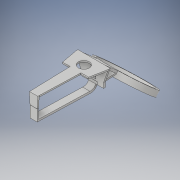
# Autodesk Inventor part: WesRoboticsInvention2019
Saved by Autodesk Inventor 2017 (Build 210142000, 142)
## iProperties
Created: 2019-11-21
Part Number: WesRoboticsInvention2019
Material: Generic
Document SubType Name: Modeling
Designer: Wes
Density: 1 g/cm^3
Appearance: Default
Author: Wes
Autodesk Inventor part; units mm, degrees
ref_plane "YZ Plane" through (0, 0, 0) normal (1, 0, 0) x (0, 1, 0)
ref_plane "XZ Plane" through (0, 0, 0) normal (0, 1, 0) x (-1, 0, 0)
ref_plane "XY Plane" through (0, 0, 0) normal (0, 0, 1) x (1, 0, 0)
sketch "sketch1 - front_main" plane through (0, 0, 0) normal (0, 0, 1) x (1, 0, 0)
  line L0 (0, 0.4311) -> (0, 247.3755) construction
  line L1 (0, 247.3755) -> (246.9445, 247.3755) construction
  line L2 (246.9445, 247.3755) -> (246.9445, 0.4311) construction
  line L3 (246.9445, 0.4311) -> (0, 0.4311) construction
  line L4 (150.2802, 116.2764) -> (77.9266, 114.0849)
  line L5 (77.9266, 114.0849) -> (77.9266, 100.4804)
  line L6 (77.9266, 100.4804) -> (48.3439, 94.9879)
  line L7 (150.2802, 131.1589) -> (77.9266, 133.3504)
  line L8 (77.9266, 133.3504) -> (77.9266, 146.9549)
  line L9 (77.9266, 146.9549) -> (48.3439, 152.4474)
  line L10 (150.2802, 116.2764) -> (150.2802, 131.1589)
  line L11 (48.3439, 94.9879) -> (48.3439, 152.4474)
  circle A0 centre (63.1352, 123.7176) radius 9.6612
  point P0 (0, 0)
  constraints: 16 end point, 1 centre point, 1 vertical, 2 other
extrude "Extrusion2" add sketch "sketch1 - front_main" along normal blind 2.5 contours L4 L5 L6 L11 L9 L8 L7 L10 | A0
sketch "sketch2 - bottom_front_tab" plane through (150.2802, 116.2764, 0) normal (1, 0, 0) x (0, 0, -1)
  line L0 (-2.5, 0) -> (-2.5, 14.8824)
  line L1 (-2.5, 0) -> (17.4726, 1.0467)
  line L2 (-2.5, 14.8824) -> (17.4726, 13.8357)
  line L3 (17.4726, 13.8357) -> (17.4726, 1.0467)
  point P0 (0, -116.2764)
  dimension "d14" = 20
  dimension "d16" = 20
  constraints: 8 end point
  measures "d14" distance of L0.start L1.end
  measures "d16" distance of L0.end L2.end
extrude "Extrusion3" add sketch "sketch2 - bottom_front_tab" along normal blind 2.5
sketch "sketch3 - top_tab" plane through (48.3439, 94.9879, 0) normal (-1, 0, 0) x (0, 0, 1)
  line L0 (30.1774, 130.7193) -> (30.1774, -83.6008) construction
  line L1 (30.1774, -83.6008) -> (-73.7679, -83.6008) construction
  line L2 (-73.7679, -83.6008) -> (-73.7679, 130.7193) construction
  line L3 (-73.7679, 130.7193) -> (30.1774, 130.7193) construction
  line L4 (2.5, 0) -> (2.5, 5.4925) projected
  line L5 (2.5, 57.4594) -> (2.5, 0)
  line L6 (2.5, 0) -> (-22.0835, 8.4648)
  line L7 (2.5, 57.4594) -> (2.5, 0) projected
  line L8 (2.5, 57.4594) -> (-22.0835, 48.9947)
  line L9 (2.5, 57.4594) -> (28.5, 57.4594) construction
  line L10 (-22.0835, 48.9947) -> (-31.0835, 48.9947)
  line L11 (-31.0835, 8.4648) -> (-22.0835, 8.4648)
  line L12 (-23.2529, 28.8344) -> (-23.2529, 35.3344)
  line L13 (-23.2529, 35.3344) -> (-17.4726, 35.1242)
  line L14 (-23.2529, 28.8344) -> (-23.2529, 22.3344)
  line L15 (-17.4726, 22.3352) -> (-17.4726, 35.1242) projected
  line L16 (-17.4726, 35.1242) -> (-17.4726, 22.3352)
  line L17 (-17.4726, 22.3352) -> (-23.2529, 22.3344)
  line L18 (-31.0835, 37.7297) -> (-31.0835, 48.9947)
  line L19 (-31.0835, 19.7297) -> (-31.0835, 8.4648)
  line L20 (-31.0835, 19.7297) -> (-26.3187, 19.7297)
  line L21 (-26.3187, 19.7297) -> (-26.3187, 37.7297)
  line L22 (-26.3187, 37.7297) -> (-31.0835, 37.7297)
  dimension "d66" = 26
  dimension "d67" = 71
  dimension "d68" = 26
  dimension "d69" = 161
  dimension "d70" = 9
  dimension "d73" = 6.5
  dimension "d74" = 6.5
  constraints: 32 end point, 4 horizontal, 2 collinear, 2 vertical, 1 equal length, 1 perpendicular, 2 other
  measures "d66" distance of L4.start L6.end
  measures "d67" angle of L5 L6
  measures "d68" distance of L5.start L8.end
  measures "d69" angle of L8 L9
  measures "d70" distance of L8.end L10.end
  measures "d73" distance of L12.start L12.end
  measures "d74" distance of L12.start L14.end
extrude "Extrusion5" add sketch "sketch3 - top_tab" along normal blind 3.5
ref_plane "Work Plane1" through (203.0833, 123.7176, 2.5) normal (0, 1, 0) x (0, 0, 1)
sketch "sketch4 - xbox_hole" plane through (0, 0, 2.5) normal (0, 0, 1) x (1, 0, 0)
  circle A0 centre (63.1352, 123.7176) radius 9.6612
  point P0 (0, 0)
  constraints: 1 centre point
extrude "Extrusion6" cut sketch "sketch4 - xbox_hole" against normal blind 2.5
sketch "sketch5 - bottom_hinge" plane through (203.0833, 123.7176, 2.5) normal (0, 1, 0) x (0, 0, 1)
  arc A0 (-39.5904, -144.1522) -> (-33.5835, -154.7394) centre (-29.9996, -145.7083) ccw
  arc A1 (-43.3245, -144.1522) -> (-33.5835, -158.2394) centre (-30.6296, -145.7854) ccw
  line L0 (-33.5835, -154.7394) -> (-33.5835, -158.2394)
  line L1 (-39.5904, -144.1522) -> (-37.1535, -52.8031)
  line L2 (-37.1535, -52.8031) -> (-20.1535, -52.8031)
  line L3 (-20.1535, -52.8031) -> (-20.1535, -50.3031)
  line L4 (0, -50.3031) -> (-19.9726, -50.3031) projected
  line L5 (-43.3245, -144.1522) -> (-40.3948, -50.3031)
  line L6 (-40.3948, -50.3031) -> (-20.1535, -50.3031)
  dimension "d82" = 17
  constraints: 12 end point, 4 point on circle, 2 centre point, 1 horizontal, 1 perpendicular, 1 vertical
  measures "d82" distance of L1.end L2.end
extrude "Extrusion7" add sketch "sketch5 - bottom_hinge" along normal mid plane 12.789
sketch "sketch6 - hinge_part" plane through (44.8439, 94.9879, 0) normal (-1, 0, 0) x (0, 0, 1)
  line L0 (-31.0835, 35.1242) -> (-31.0835, 37.6242)
  line L1 (-31.0835, 37.6242) -> (-26.4835, 37.6242)
  line L2 (-31.0835, 22.3352) -> (-31.0835, 19.8352)
  line L3 (-31.0835, 35.1242) -> (-31.0835, 22.3352)
  line L4 (-31.0835, 19.8352) -> (-26.4835, 19.8352)
  line L5 (-26.4835, 19.8352) -> (-26.4835, 37.6242)
  dimension "d92" = 2.5
  dimension "d94" = 4.6
  dimension "d95" = 2.5
  constraints: 12 end point, 2 horizontal, 2 vertical, 1 collinear, 1 perpendicular
  measures "d92" distance of L0.start L0.end
  measures "d94" distance of L0.end L1.end
  measures "d95" distance of L2.start L2.end
extrude "Extrusion8" add sketch "sketch6 - hinge_part" against normal blind 3.5
sketch "sketch7 - drink_arm" plane through (203.0833, 123.7176, 2.5) normal (0, 1, 0) x (0, 0, 1)
  line L0 (0, -158.2394) -> (-21.4626, -182.9294)
  line L1 (0, -158.2394) -> (32.7145, -158.2394) construction
  line L2 (-21.4626, -182.9294) -> (-24.4815, -180.3051)
  line L3 (0, -158.2394) -> (-5.3001, -158.2394)
  line L4 (-24.4815, -180.3051) -> (-25.7529, -158.2394)
  line L5 (-22.9721, -158.2394) -> (-21.8735, -177.305)
  line L6 (-5.3001, -158.2394) -> (-21.8735, -177.305)
  line L7 (-22.9721, -158.2394) -> (-25.7529, -158.2394)
  dimension "d98" = 131
  dimension "d99" = 4
  constraints: 16 end point, 2 horizontal, 1 equal length, 1 perpendicular
  measures "d98" angle of L0 L1
  measures "d99" distance of L0.end L2.end
extrude "Extrusion9" add sketch "sketch7 - drink_arm" along normal mid plane 38
sketch "sketch8 - support_arm_arc_hole" plane through (25.7783, 104.7176, -19.3735) normal (0.057524, 0, 0.9983441) x (0.9983441, 0, -0.057524)
  line L0 (19.1574, 4.5062) -> (19.1574, 33.5009)
  arc A0 (19.1574, 33.5009) -> (19.1574, 4.5062) centre (20.5085, 19.0036) ccw
  point P0 (-26.8501, -104.7176)
  constraints: 2 end point, 2 point on circle, 1 centre point
extrude "Extrusion10" cut sketch "sketch8 - support_arm_arc_hole" against normal blind 10
sketch "sketch9 - cup_holder" plane through (44.8439, 104.7176, 2.5) normal (-0.656059, 0, 0.7547096) x (0.7547096, 0, 0.656059)
  line L0 (-32.7145, 19) -> (-75.4429, 19) construction
  circle A0 centre (-75.4429, 19) radius 42.7285
  circle A1 centre (-75.4429, 19) radius 48.0116
  constraints: 2 coincident, 2 end point, 1 centre point, 1 horizontal, 1 horizontal alignment, 2 other
extrude "Extrusion11" add sketch "sketch9 - cup_holder" against normal blind 10
body "Solid2"
